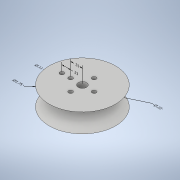
# Autodesk Inventor part: String Little Big Wheel V4
Saved by Autodesk Inventor 2020 (Build 240168000, 168)
## iProperties
Created: 2020-01-07
Part Number: String Little Big Wheel V4
Material: Generic
Document SubType Name: Modeling
Designer: AOFUser
Density: 1 g/cm^3
Appearance: Default
Author: AOFUser
Autodesk Inventor part; units mm, degrees
ref_plane "YZ Plane" through (0, 0, 0) normal (1, 0, 0) x (0, 1, 0)
ref_plane "XZ Plane" through (0, 0, 0) normal (0, 1, 0) x (-1, 0, 0)
ref_plane "XY Plane" through (0, 0, 0) normal (0, 0, 1) x (1, 0, 0)
sketch "Sketch1" plane through (0, 0, 0) normal (0, 1, 0) x (-1, 0, 0)
  circle A0 centre (0, 0) radius 22.225
  dimension "d0" = 44.45
  constraints: 1 centre point, 1 coincident
  measures "d0" diameter of A0
extrude "Extrusion1" add sketch "Sketch1" along normal blind 6.35
chamfer "Chamfer1" distance 12.7 distance2 6.35 1 edges at (22.225, 6.35, 0) measured on face at (21.725, 6.35, 0)
sketch "Sketch2" plane through (0, 6.35, 0) normal (0, 1, 0) x (1, 0, 0)
  circle A0 centre (0, 0) radius 22.225
  dimension "d57" = 44.45
  constraints: 1 centre point, 1 coincident
  measures "d57" diameter of A0
extrude "Extrusion2" add sketch "Sketch2" along normal blind 6.35
chamfer "Chamfer2" distance 12.7 distance2 6.35 1 edges at (-22.225, 6.35, 0) measured on face at (-21.725, 6.35, 0)
sketch "Sketch4" plane through (0, 12.7, 0) normal (0, 1, 0) x (1, 0, 0)
  circle A0 centre (0, 0) radius 2.794
  line L0 (0, 0) -> (-7.874, 0)
  line L1 (-7.874, 0) -> (-13.716, 0)
  line L2 (0, 0) -> (0, 7.874)
  line L3 (0, 0) -> (7.874, 0)
  line L4 (0, 0) -> (0, -7.874)
  circle A1 centre (0, -7.874) radius 1.397
  circle A2 centre (7.874, 0) radius 1.397
  circle A3 centre (0, 7.874) radius 1.397
  circle A4 centre (-7.874, 0) radius 1.397
  circle A5 centre (-13.716, 0) radius 1.397
  dimension "d28" = 5.588
  dimension "d29" = 7.874
  dimension "d30" = 5.842
  dimension "d31" = 7.874
  dimension "d32" = 7.874
  dimension "d33" = 7.874
  dimension "d34" = 2.794
  dimension "d35" = 2.794
  dimension "d36" = 2.794
  dimension "d37" = 2.794
  dimension "d38" = 2.794
  constraints: 10 end point, 6 centre point, 6 coincident, 2 horizontal, 2 vertical, 1 point on line
  measures "d28" diameter of A0
  measures "d29" distance of L0.start L0.end
  measures "d30" distance of L0.end L1.end
  measures "d31" distance of L0.start L2.end
  measures "d32" distance of L0.start L3.end
  measures "d33" distance of L0.start L4.end
  measures "d34" diameter of A1
  measures "d35" diameter of A2
  measures "d36" diameter of A3
  measures "d37" diameter of A4
  measures "d38" diameter of A5
extrude "Extrusion3" cut sketch "Sketch4" against normal blind 15.24
sketch "Sketch5" plane through (0, 0, 0) normal (0, -1, 0) x (1, 0, 0)
  circle A0 centre (0, 0) radius 2.794 projected
  circle A1 centre (0, 0) radius 11.1125
  dimension "d58" = 22.225
  constraints: 1 centre point, 1 coincident
  measures "d58" diameter of A1
extrude "Extrusion4" cut sketch "Sketch5" against normal blind 5.08
body "Solid1"
